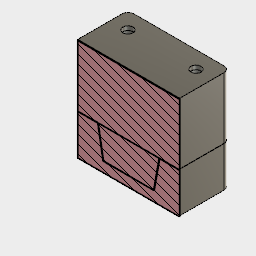
Leg_Extensions_v8 (Autodesk Fusion 360 design; units mm, degrees)
Autodesk Fusion 360 part; units mm, degrees
sketch "Main" plane through (0, 0, 0) normal (0, 0, 1) x (1, 0, 0) in component "Lower Leg"
  line L0 (25.25, 25.25) -> (-25.25, 25.25)
  line L1 (-25.25, 25.25) -> (-25.25, -25.25)
  line L2 (-25.25, -25.25) -> (25.25, -25.25)
  line L3 (25.25, -25.25) -> (25.25, 25.25)
  line L4 (25.25, 25.25) -> (-25.25, -25.25) construction
  line L5 (-25.25, 25.25) -> (25.25, -25.25) construction
  dimension "d5" = 50.5
  dimension "d6" = 50.5
  constraint perpendicular L0 L1
  constraint parallel L0 L2
  constraint parallel L1 L3
  constraint horizontal L0
  constraint coincident L4 origin
  constraint coincident L5 origin
extrude "Extrude1" add sketch "Main" along normal blind 20 makes body 1 in component "Lower Leg"
ref_plane "WorkPlane1" through (0, 0, 10) normal (0, -1, 0) x (1, 0, 0) in component "Lower Leg"
sketch "Cone" plane through (0, 0, 10) normal (0, -1, 0) x (1, 0, 0) in component "Lower Leg"
  line L0 (25.25, 10) -> (-25.25, 10)
  line L1 (-25.25, 10) -> (25.25, 10)
  line L2 (0, 10) -> (15.25, 10)
  line L3 (12.6051, -5) -> (0, -5)
  line L4 (0, -5) -> (0, 10)
  line L5 (15.25, 10) -> (12.6051, -5)
  dimension "d11" = 15
  dimension "d14" = 80
  dimension "d16" = 15.25
  constraint midpoint L0 origin
  constraint coincident L1 origin
  constraint parallel L0 L3
  constraint perpendicular L0 L4
  measures "d14" angle of L2 L5
revolve "Revolve1" cut sketch "Cone" angle 360 about axis through (0, 0, 1.75) along (0, 0, 1) bodies 1 in component "Lower Leg"
sketch "Mounting Holes" plane through (0, 0, 20) normal (0, 0, 1) x (-1, 0, 0) in component "Lower Leg"
  circle A0 centre (0, 0) radius 15.25
  line L0 (-25.25, 25.25) -> (-25.25, -25.25)
  line L1 (-25.25, -25.25) -> (25.25, -25.25)
  line L2 (25.25, -25.25) -> (25.25, 25.25)
  line L3 (25.25, 25.25) -> (-25.25, 25.25)
  circle A1 centre (16.8333, -16.8333) radius 2.5
  line L4 (-25.25, -25.25) -> (-25.25, 25.25)
  line L5 (-25.25, 25.25) -> (25.25, 25.25)
  line L6 (25.25, 25.25) -> (25.25, -25.25)
  line L7 (25.25, -25.25) -> (-25.25, -25.25)
  circle A2 centre (16.8333, -16.8333) radius 5
  dimension "d18" = 5
  dimension "d21" = 8.4167
  dimension "d23" = 8.4167
  dimension "d24" = 10
  constraint concentric A1 A2
  measures "d18" diameter of A1
  measures "d24" diameter of A2
extrude "Extrude2" cut sketch "Mounting Holes" against normal up to surface (20 mm away) contours A1 bodies 1 in component "Lower Leg"
extrude "Extrude3" cut sketch "Mounting Holes" against normal blind 18 contours A2 bodies 1 in component "Lower Leg"
pattern_circular "C-Pattern1" count 4 over 360 about axis through (0, 0, 20) along (0, 0, -1) of "Extrude2", "Extrude3" in component "Lower Leg"
fillet "Fillet1" radius 3 4 edges at (-25.25, 25.25, 10) (-25.25, -25.25, 10) (25.25, -25.25, 10) (25.25, 25.25, 10) on bodies 1 in component "Lower Leg"
ref_plane "WorkPlane1" through (0, 0, 20.1) normal (0, 0, 1) x (1, 0, 0) in component "Upper Leg"
sketch "Body and Mounting" plane through (0, 0, 20.1) normal (0, 0, 1) x (1, 0, 0) in component "Upper Leg"
  arc A0 (25.25, 22.25) -> (22.25, 25.25) centre (22.25, 22.25) ccw
  line L0 (22.25, 25.25) -> (-22.25, 25.25)
  line L1 (25.25, -22.25) -> (25.25, 22.25)
  arc A1 (22.25, -25.25) -> (25.25, -22.25) centre (22.25, -22.25) ccw
  line L2 (-22.25, -25.25) -> (22.25, -25.25)
  arc A2 (-25.25, -22.25) -> (-22.25, -25.25) centre (-22.25, -22.25) ccw
  line L3 (-25.25, 22.25) -> (-25.25, -22.25)
  arc A3 (-22.25, 25.25) -> (-25.25, 22.25) centre (-22.25, 22.25) ccw
  line L4 (22.25, -25.25) -> (-22.25, -25.25)
  line L5 (-22.25, -25.25) -> (22.25, -25.25)
  circle A4 centre (-16.8333, -16.8333) radius 5
  circle A5 centre (-16.8333, -16.8333) radius 5
  circle A6 centre (-16.8333, -16.8333) radius 5
  circle A7 centre (-16.8333, -16.8333) radius 2.5
  arc A8 (25.25, 22.25) -> (22.25, 25.25) centre (22.25, 22.25) ccw
  line L6 (25.25, 22.25) -> (25.25, -22.25)
  arc A9 (22.25, -25.25) -> (25.25, -22.25) centre (22.25, -22.25) ccw
  line L7 (22.25, -25.25) -> (-22.25, -25.25)
  arc A10 (-25.25, -22.25) -> (-22.25, -25.25) centre (-22.25, -22.25) ccw
  line L8 (-25.25, -22.25) -> (-25.25, 22.25)
  arc A11 (-22.25, 25.25) -> (-25.25, 22.25) centre (-22.25, 22.25) ccw
  line L9 (-22.25, 25.25) -> (22.25, 25.25)
  circle A12 centre (-16.8333, -16.8333) radius 5
extrude "Extrude1'" add sketch "Body and Mounting" along normal blind 30.3 separate body contours A0 L0 L1 A1 L2 A2 L3 A3 L4 L5 A8 L6 A9 L7 A10 L8 A11 L9 | A4 A5 A6 A12 | A7 makes body 2 in component "Upper Leg"
extrude "Extrude2'" cut sketch "Body and Mounting" along normal up to surface (30.3 mm away) contours A7 bodies 2 in component "Upper Leg"
extrude "Extrude3'" cut sketch "Body and Mounting" along normal blind 28.3 contours A4 A5 A6 A12 bodies 2 in component "Upper Leg"
ref_plane "WorkPlane2" through (0, 0, 35.25) normal (0, -1, 0) x (1, 0, 0) in component "Upper Leg"
ref_plane "WorkPlane3" through (0, 0, 35.25) normal (1, 0, 0) x (0, 1, 0) in component "Upper Leg"
pattern_circular "C-Pattern1'" count 4 over 360 about axis through (0, 0, 60.45) along (0, 0, -1) of 2 faces at (-11.8395, -17.0826, 38.9667) (-12.6946, -17.2059, 48.4) on bodies 2 in component "Upper Leg"
pattern_circular "C-Pattern2" count 4 over 360 about axis through (0, 0, 60.45) along (0, 0, -1) of 1 faces at (-14.3458, -17.0823, 49.7333) on bodies 2 in component "Upper Leg"
sketch "Cone (2)" plane through (0, 0, 35.2) normal (0, -1, 0) x (1, 0, 0) in component "Upper Leg"
  line L0 (0, -15.1) -> (15.15, -15.1)
  line L1 (15.15, -15.1) -> (12.5051, -30.1)
  line L2 (25.25, -15.2) -> (-25.25, -15.2)
  line L3 (12.5051, -30.1) -> (0, -30.1)
  line L4 (0, -30.1) -> (0, -15.1)
  dimension "d47" = 80
  dimension "d48" = 15.15
  dimension "d51" = 15
  constraint parallel L2 L3
  constraint parallel L0 L3
  constraint perpendicular L0 L4
  measures "d47" angle of L0 L1
revolve "Revolve2" add sketch "Cone (2)" angle 360 about axis through (0, 0, 60.45) along (0, 0, -1) separate body makes body 3 in component "Upper Leg"
component "Lower Leg" placed x (1, 0, 0) y (0, 1, 0) z (0, 0, 1) at (0, 0, 0)
component "Upper Leg" placed x (1, 0, 0) y (0, 1, 0) z (0, 0, 1) at (0, 0, 0)
equation "legwidth = 50.5 mm"
equation "totheight = 50.3 mm"
equation "botheight = 20 mm"
equation "topheight = totheight - botheight"
equation "d5 = legwidth"
equation "d6 = legwidth"
equation "d7 = botheight"
equation "coneheight = botheight - 5 mm"
equation "conegap = 0.1 mm"
equation "d11 = coneheight"
equation "conerad = ( legwidth / 2 ) - 10 mm"
equation "d14 = coneang"
equation "coneang = 80 deg"
equation "d16 = conerad"
equation "d18 = mountscrewhole"
equation "mountscrewhead = 10 mm"
equation "mountscrewhole = 5 mm"
equation "d21 = holedistance"
equation "holedistance = legwidth / 6"
equation "d23 = holedistance"
equation "d24 = mountscrewhead"
equation "mountscrewthickness = 2 mm"
equation "d28 = -( botheight - mountscrewthickness )"
equation "d32 = legfillet"
equation "legfillet = 3 mm"
equation "d34 = vertical_gap"
equation "vertical_gap = 0.1 mm"
equation "d36 = topheight"
equation "d40 = ( topheight - mountscrewthickness )"
equation "d47 = coneang"
equation "d48 = conerad - conegap"
equation "d51 = coneheight"
